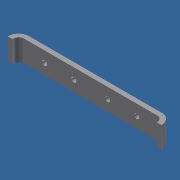
# Autodesk Inventor part: LAMINA
Saved by Autodesk Inventor 2012 SP1 (Build 160190100, 190)
## iProperties
Created: 2012-07-23
Part Number: LAMINA
Material: Default
Document SubType Name: Modeling
Designer: bruno.silveira
Density: 1 g/cm^3
Author: bruno.silveira
Autodesk Inventor part; units mm, degrees
ref_plane "YZ Plane" through (0, 0, 0) normal (1, 0, 0) x (0, 1, 0)
ref_plane "XZ Plane" through (0, 0, 0) normal (0, 1, 0) x (-1, 0, 0)
ref_plane "XY Plane" through (0, 0, 0) normal (0, 0, 1) x (1, 0, 0)
sketch "Sketch1" plane through (0, 0, 0) normal (0, 0, 1) x (1, 0, 0)
  line L0 (100, 0.14) -> (100, 0)
  line L1 (0, 0.14) -> (0, 0)
  arc A0 (96.9975, 0) -> (94, 4) centre (93.0167, 0.14) ccw
  arc A1 (100, 0.14) -> (94.323, 7) centre (93.0167, 0.14) ccw
  arc A2 (6, 4) -> (3.0025, 0) centre (6.9833, 0.14) ccw
  arc A3 (5.677, 7) -> (0, 0.14) centre (6.9833, 0.14) ccw
  line L2 (5.677, 7) -> (94.323, 7)
  line L3 (96.9975, 0) -> (100, 0)
  line L4 (6, 4) -> (94, 4)
  line L5 (3, 0.14) -> (3, 0)
  line L6 (0, 0) -> (3.0025, 0)
  dimension "d0" = 100
  dimension "d6" = 3
  dimension "d7" = 7
  dimension "d8" = 3
  constraints: 14 end point, 9 point on circle, 4 centre point, 4 parallel, 2 perpendicular, 1 horizontal
  measures "d0" distance of L1.end L0.end
  measures "d6" radial gap between concentric circles of A0 A1
  measures "d7" distance between parallel lines of L3 L2
  measures "d8" radial gap between concentric circles of A3 A2
extrude "Extrusion1" add sketch "Sketch1" along normal blind 14
sketch "Sketch2" plane through (5.677, 7, 0) normal (0, 1, 0) x (1, 0, 0)
  line L0 (0, -14) -> (88.6461, -14) projected
  line L1 (0, 0) -> (88.6461, 0) projected
  line L2 (44.323, 0) -> (44.323, -14)
  point P0 (-5.677, 0)
  point P1 (14.323, -7)
  point P2 (33.323, -7)
  point P3 (55.323, -7)
  point P4 (74.323, -7)
  dimension "d11" = 22
  dimension "d12" = 60
  dimension "d13" = 11
  dimension "d14" = 30
  dimension "d15" = 7
  constraints: 2 end point, 2 midpoint
  measures "d11" distance of point (55.323, -7) point (33.323, -7)
  measures "d12" distance of point (74.323, -7) point (14.323, -7)
  measures "d13" distance from line of L2 point (33.323, -7)
  measures "d14" distance from line of L2 point (14.323, -7)
  measures "d15" distance from line of L0 point (74.323, -7)
hole "Hole1" at (20, 7, 7) at (39, 7, 7) at (61, 7, 7) at (80, 7, 7) direction (0, -1, 0) diameter 3.2 depth 3 tip angle 118
body "Solid1"
